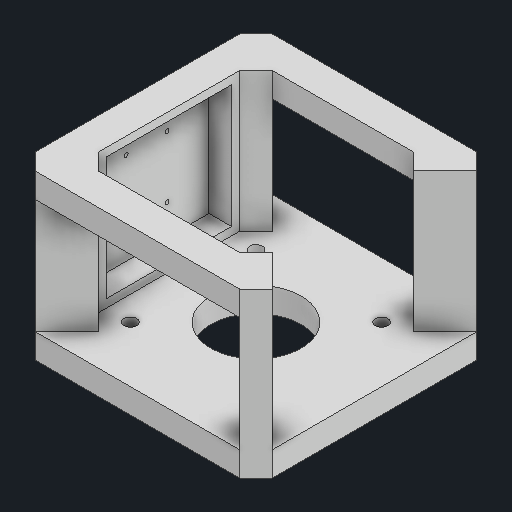
# Autodesk Inventor part: table_motor_mount
Saved by Autodesk Inventor 2025 (Build 290162010, 162A)
## iProperties
Created: 2024-07-08
Part Number: table_motor_mount
Material: Generic
Document SubType Name: Modeling
Designer: mihir
Density: 1 g/cm^3
Appearance: Default
Author: mihir
Autodesk Inventor part; units mm, degrees
ref_plane "YZ Plane" through (0, 0, 0) normal (1, 0, 0) x (0, 1, 0)
ref_plane "XZ Plane" through (0, 0, 0) normal (0, 1, 0) x (-1, 0, 0)
ref_plane "XY Plane" through (0, 0, 0) normal (0, 0, 1) x (1, 0, 0)
sketch "Sketch1" plane through (0, 0, 0) normal (0, 1, 0) x (-1, 0, 0)
  circle A0 centre (0, 0) radius 11.05
  line L0 (21.25, 17.25) -> (21.25, -17.25)
  line L1 (21.25, -17.25) -> (17.25, -21.25)
  line L2 (17.25, -21.25) -> (-17.25, -21.25)
  line L3 (-17.25, -21.25) -> (-21.25, -17.25)
  line L4 (-21.25, -17.25) -> (-21.25, 17.25)
  line L5 (-21.25, 17.25) -> (-17.25, 21.25)
  line L6 (-17.25, 21.25) -> (17.25, 21.25)
  line L7 (17.25, 21.25) -> (21.25, 17.25)
  line L8 (21.25, 0) -> (-21.25, 0) construction
  line L9 (0, 21.25) -> (0, -21.25) construction
  circle A1 centre (15.3506, -15.3506) radius 1.55
  line L10 (15.3506, -15.3506) -> (0, 0) construction
  circle A2 centre (15.3506, 15.3506) radius 1.55
  circle A3 centre (-15.3506, 15.3506) radius 1.55
  circle A4 centre (-15.3506, -15.3506) radius 1.55
  point P0 (0, 0)
  dimension "d0" = 22.1
  dimension "d1" = 135
  dimension "d2" = 42.5
  dimension "d3" = 5.6569
  dimension "d25" = 3.1
  dimension "d26" = 21.709
  dimension "d27" = 45
  dimension "d30" = 360
  constraints: 22 end point, 8 perpendicular, 6 midpoint, 5 centre point, 2 coincident, 2 parallel, 1 vertical, 9 other
  measures "d0" diameter of A0
  measures "d2" distance between parallel lines of L2 L6
  measures "d3" distance of L6.end L0.start
  measures "d25" diameter of A1
  measures "d26" distance of L10.start L10.end
extrude "Extrusion1" add sketch "Sketch1" along normal blind 6
sketch "Sketch6" plane through (0, 0, 0) normal (0, -1, 0) x (1, 0, 0)
  line L0 (29, -25) -> (29, 25)
  line L1 (29, 25) -> (25, 29)
  line L2 (25, 29) -> (-25, 29)
  line L3 (-25, 29) -> (-29, 25)
  line L4 (-29, 25) -> (-29, -25)
  line L5 (-29, -25) -> (-25, -29)
  line L6 (-25, -29) -> (25, -29)
  line L7 (25, -29) -> (29, -25)
  line L8 (27, -27) -> (-27, 27) construction
  line L9 (-17.25, 21.25) -> (17.25, 21.25) construction
  line L10 (25, 29) -> (17.25, 21.25) construction
  line L11 (29, 25) -> (21.25, 17.25) construction
  line L12 (21.25, -17.25) -> (17.25, -21.25) projected
  line L13 (21.25, 17.25) -> (21.25, -17.25) projected
  line L14 (21.25, -17.25) -> (21.25, 17.25)
  line L15 (17.25, 21.25) -> (21.25, 17.25) projected
  line L16 (21.25, 17.25) -> (17.25, 21.25)
  line L17 (17.25, 21.25) -> (-17.25, 21.25)
  line L18 (-21.25, 17.25) -> (-17.25, 21.25) projected
  line L19 (-21.25, 17.25) -> (-17.25, 21.25)
  line L20 (17.25, 21.25) -> (21.25, 17.25)
  line L21 (-21.25, -17.25) -> (-21.25, 17.25) projected
  line L22 (-21.25, 17.25) -> (-21.25, -17.25)
  line L23 (-21.25, -17.25) -> (-17.25, -21.25)
  line L24 (-17.25, -21.25) -> (17.25, -21.25)
  line L25 (17.25, -21.25) -> (21.25, -17.25)
  point P0 (0, 0)
  point P1 (0, 0)
  dimension "d32" = 135
  dimension "d33" = 135
  dimension "d34" = 50
  constraints: 40 end point, 9 perpendicular, 8 equal length, 3 midpoint, 2 point on line, 1 coincident, 1 vertical
  measures "d34" distance of L0.start L0.end
extrude "Extrusion5" add sketch "Sketch6" against normal blind 40
sketch "Sketch8" plane through (0, 40, 0) normal (0, 1, 0) x (1, 0, 0)
  line L0 (29, -25) -> (29, 25) projected
  line L1 (21.25, -17.25) -> (21.25, 17.25) projected
  line L2 (29, 25) -> (21.25, 17.25)
  line L3 (17.25, -21.25) -> (21.25, -17.25) projected
  line L4 (21.25, 17.25) -> (21.25, -17.25)
  line L5 (21.25, -17.25) -> (29, -25)
  line L6 (29, -25) -> (29, 25)
  point P0 (0, 0)
  constraints: 8 end point, 1 parallel, 1 perpendicular, 1 vertical
extrude "Extrusion6" cut sketch "Sketch8" against normal blind 34
sketch "Sketch9" plane through (0, 6, 0) normal (0, 1, 0) x (1, 0, 0)
  line L0 (25, 29) -> (-25, 29) projected
  line L1 (17.25, 21.25) -> (21.25, 17.25) projected
  line L2 (25, 29) -> (17.25, 21.25)
  line L3 (-21.25, 17.25) -> (-17.25, 21.25) projected
  line L4 (17.25, 21.25) -> (-17.25, 21.25)
  line L5 (-17.25, 21.25) -> (-25, 29)
  line L6 (-25, 29) -> (25, 29)
  line L7 (-17.25, -21.25) -> (17.25, -21.25) projected
  line L8 (25, -29) -> (-25, -29) projected
  line L9 (17.25, -21.25) -> (25, -29)
  line L10 (25, -29) -> (-25, -29)
  line L11 (-25, -29) -> (-17.25, -21.25)
  line L12 (-17.25, -21.25) -> (17.25, -21.25)
  point P0 (0, 0)
  constraints: 16 end point, 3 perpendicular, 2 parallel, 1 collinear, 1 horizontal
extrude "Extrusion7" cut sketch "Sketch9" along normal blind 28
sketch "Sketch10" plane through (-21.25, 6, -17.25) normal (1, 0, 0) x (0, 0, -1)
  line L0 (7.75, 0) -> (-42.25, 0) construction
  line L1 (-17.25, 0) -> (-17.25, 34) construction
  line L2 (-34.5, 34) -> (0, 34) construction
  line L3 (0, 0) -> (0, 34) construction
  line L4 (0, 17) -> (-34.5, 17) construction
  line L5 (-34.5, 0) -> (-34.5, 34) construction
  line L6 (-32.5, 2) -> (-2, 2)
  line L7 (-2, 2) -> (-2, 32)
  line L8 (-2, 32) -> (-32.5, 32)
  line L9 (-32.5, 32) -> (-32.5, 2)
  line L10 (-17.25, 2) -> (-17.25, 32) construction
  line L11 (-32.5, 17) -> (-2, 17) construction
  point P0 (-17.25, -6)
  point P1 (-17.25, 17)
  dimension "d41" = 2
  dimension "d42" = 2
  constraints: 16 end point, 10 midpoint, 2 parallel, 1 horizontal, 1 perpendicular
  measures "d41" distance between parallel lines of L0 L6
  measures "d42" distance between parallel lines of L3 L7
extrude "Extrusion8" cut sketch "Sketch10" against normal blind 5.5
sketch "Sketch11" plane through (-26.75, 6, -17.25) normal (1, 0, 0) x (0, 0, -1)
  line L0 (-12.25, 9.5) -> (-22.25, 9.5) construction
  line L1 (-22.25, 9.5) -> (-22.25, 24.5) construction
  line L2 (-22.25, 24.5) -> (-12.25, 24.5) construction
  line L3 (-12.25, 24.5) -> (-12.25, 9.5) construction
  line L4 (-2, 32) -> (-2, 2) construction
  line L5 (-32.5, 2) -> (-32.5, 32) construction
  line L6 (-2, 2) -> (-32.5, 32) construction
  line L7 (-32.5, 32) -> (-2, 32) construction
  line L8 (-32.5, 2) -> (-2, 32) construction
  line L9 (-12.25, 9.5) -> (-22.25, 24.5) construction
  line L10 (-22.25, 9.5) -> (-12.25, 24.5) construction
  point P0 (-17.25, -6)
  point P1 (-17.25, 17)
  dimension "d45" = 10
  dimension "d46" = 15
  constraints: 16 end point, 4 coincident, 2 midpoint, 2 parallel, 1 horizontal, 1 perpendicular
  measures "d45" distance of L1.end L2.end
  measures "d46" distance of L0.end L1.end
hole "Hole2" at (-26.75, 15.5, -5) at (-26.75, 15.5, 5) at (-26.75, 30.5, -5) at (-26.75, 30.5, 5) direction (-1, 0, 0) diameter 1 depth 2.25 tip angle 118
equation "\"d0\" = shaft_hole_diameter"
equation "\"d4\" = mount_face_thickness"
equation "\"d34\" = mount_width"
equation "\"d35\" = mount_length"
equation "\"d37\" = mount_length - mount_face_thickness"
equation "\"d39\" = mount_length - 2 * mount_face_thickness"
equation "\"d45\" = screw_x"
equation "\"d46\" = screw_y"
equation "\"d47\" = screw_diameter"
equation "\"shaft_hole_diameter\" = 22.1"
equation "\"mount_width\" = 50"
equation "\"mount_slant_length\" = 5"
equation "\"mount_face_thickness\" = 6"
equation "\"mount_length\" = 40"
equation "\"screw_x\" = 10"
equation "\"screw_y\" = 15"
equation "\"screw_diameter\" = 1"
body "Solid1"
